GearboxTop_v1 (Autodesk Fusion 360 design; units mm, degrees)
Autodesk Fusion 360 part; units mm, degrees
note: some values were not read from the file. Set by a fixed rule: which sketch regions a step uses.
sketch "Sketch1" plane through (0, 0, 0) normal (0, 0, 1) x (1, 0, 0)
  circle A0 centre (0, 0) radius 65
  circle A1 centre (0, 0) radius 61.0225 construction
  circle A2 centre (0, 0) radius 39.5
  circle A3 centre (0, -61.0225) radius 1.5
  dimension "d1" = 130
  dimension "d2" = 122.045
  dimension "d3" = 79
  dimension "ScrewDia" = 3
  constraint coincident A0.centre A1.centre
  constraint concentric A0 A1
  constraint coincident A1 A3.centre
  measures "d1" diameter of A0
  measures "d2" diameter of A1
  measures "d3" diameter of A2
  measures "ScrewDia" diameter of A3
extrude "Extrude1" add sketch "Sketch1" along normal blind 2 contours A0 | A3
sketch "Sketch2" plane through (0, 0, 2) normal (0, 0, 1) x (-1, 0, 0)
  circle A0 centre (0, 0) radius 39.5
  circle A1 centre (0, 0) radius 65
  circle A2 centre (0, 0) radius 42.5
  dimension "BearingDia" = 85
  constraint coincident A0.centre A1.centre
  measures "BearingDia" diameter of A2
extrude "Extrude2" add sketch "Sketch2" along normal blind 10 contours A1
extrude "Extrude3" cut sketch "Sketch1" along normal blind 25 contours A3
sketch "Sketch3" plane through (0, 0, 12) normal (0, 0, 1) x (-1, 0, 0)
  circle A0 centre (0, 61.0225) radius 1.5
  circle A1 centre (0, 0) radius 42.5
  circle A2 centre (0, 0) radius 65
  circle A3 centre (0, -61.0225) radius 2.5
  dimension "ScrewHeadDia" = 5
  measures "ScrewHeadDia" diameter of A3
extrude "Extrude4" cut sketch "Sketch3" against normal blind 5 contours A3
pattern_circular "C-Pattern1" count 6 over 360 about axis through (0, 0, 1.75) along (0, 0, 1) of "Extrude3", "Extrude4"
equation "BearingHieght = 10 mm"
equation "ScrewHeadDepth = -5 mm"
